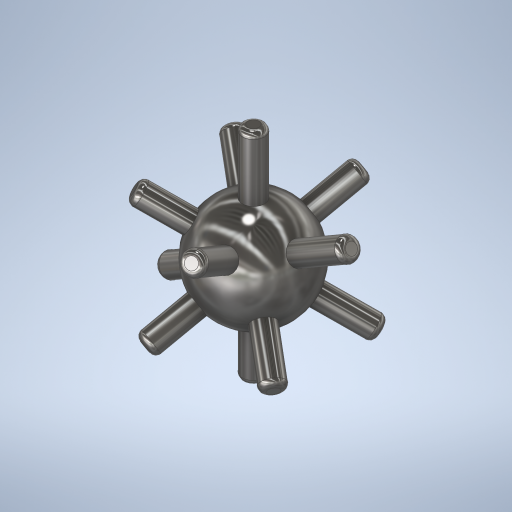
# Autodesk Inventor part: jezek v
Saved by Autodesk Inventor 2023 (Build 270158000, 158)
## iProperties
Created: 2024-01-23
Part Number: jezek v
Material: Všeobecné
Document SubType Name: Modeling
Designer: 42073
Density: 1 g/cm^3
Appearance: Ocel – leštěná
Mass: 5.1124 g
Surface Area: 25.3749 cm^2
Volume: 5.1124 cm^3
Author: 42073
Autodesk Inventor part; units mm, degrees
sketch "Náčrt1" plane through (0, 0, 0) normal (0, 0, 1) x (1, 0, 0)
  circle A0 centre (0, 0) radius 9.6
  dimension "d0" = 19.2
  constraints: 1 centre point, 1 coincident
  measures "d0" diameter of A0
extrude "Vysunutí1" add sketch "Náčrt1" along normal mid plane 19.2
fillet "Zaoblení1" radius 9.6 2 edges at (-9.6, 0, 9.6) (-9.6, 0, -9.6)
sketch "Náčrt2" plane through (0, 0, 0) normal (0, 0, 1) x (1, 0, 0)
  line L0 (0, 0) -> (20, 0)
  line L1 (0, 0) -> (6.1803, 19.0211)
  line L2 (0, 0) -> (20, 0) construction
  line L3 (0, 0) -> (-16.1803, 11.7557)
  line L4 (0, 0) -> (20, 0) construction
  line L5 (0, 0) -> (-16.1803, -11.7557)
  line L6 (0, 0) -> (20, 0) construction
  line L7 (0, 0) -> (6.1803, -19.0211)
  line L8 (0, 0) -> (20, 0) construction
  dimension "d4" = 20
  dimension "d5" = 20
  dimension "d6" = 72
  dimension "d7" = 20
  dimension "d8" = 144
  dimension "d9" = 20
  dimension "d10" = 216
  dimension "d11" = 20
  dimension "d12" = 72
  constraints: 18 end point, 5 horizontal, 4 equal length
  measures "d4" distance of L0.start L0.end
  measures "d5" distance of L0.start L1.end
  measures "d6" angle of L2 L1
  measures "d7" distance of L0.start L3.end
  measures "d8" angle of L4 L3
  measures "d9" distance of L0.start L5.end
  measures "d11" distance of L0.start L7.end
  measures "d12" angle of L7 L8
ref_plane "Pracovní rovina2" through (0, 0, 20) normal (0, 0, 1) x (1, 0, 0)
sketch "Náčrt3" plane through (0, 0, 20) normal (0, 0, 1) x (1, 0, 0)
  line L0 (0, 0) -> (6.1803, 19.0211)
  line L1 (0, 0) -> (20, 0) construction
  line L2 (0, 0) -> (-16.1803, 11.7557)
  line L3 (0, 0) -> (20, 0) construction
  line L4 (0, 0) -> (20, 0)
  line L5 (0, 0) -> (6.1803, -19.0211)
  line L6 (0, 0) -> (20, 0) construction
  line L7 (0, 0) -> (-16.1803, -11.7557)
  line L8 (0, 0) -> (20, 0) construction
  dimension "d14" = 20
  dimension "d15" = 72
  dimension "d16" = 20
  dimension "d17" = 144
  dimension "d18" = 20
  dimension "d19" = 72
  dimension "d20" = 20
  dimension "d21" = 144
  constraints: 18 end point, 4 equal length, 4 horizontal, 1 collinear
  measures "d14" distance of L0.start L0.end
  measures "d15" angle of L1 L0
  measures "d16" distance of L0.start L2.end
  measures "d17" angle of L3 L2
  measures "d18" distance of L0.start L5.end
  measures "d19" angle of L5 L6
  measures "d20" distance of L0.start L7.end
  measures "d21" angle of L7 L8
ref_plane "Pracovní rovina3" through (0, 0, 20) normal (-0.9511, 0.309, 0) x (0.309, 0.9511, 0)
sketch "Náčrt4" plane through (0, 0, 20) normal (-0.9511, 0.309, 0) x (0.309, 0.9511, 0)
  line L0 (0, 20) -> (0, 39.1)
  line L1 (0, 20) -> (15.9349, 10.8)
  line L2 (0, 20) -> (18.4, 20) construction
  line L3 (0, 20) -> (-15.7617, 29.1)
  line L4 (0, 20) -> (0, -1.1)
  dimension "d22" = 19.1
  dimension "d23" = 18.4
  dimension "d24" = 30
  dimension "d25" = 18.2
  dimension "d26" = 21.1
  constraints: 10 end point, 2 vertical, 1 equal length, 1 horizontal, 1 point on line
  measures "d22" distance of L0.start L0.end
  measures "d23" distance of L0.start L1.end
  measures "d24" angle of L1 L2
  measures "d25" distance of L0.start L3.end
  measures "d26" distance of L0.start L4.end
ref_plane "Pracovní rovina4" through (0, 0, 0) normal (0, -1, 0) x (1, 0, 0)
sketch "Náčrt5" plane through (0, 0, 0) normal (0, -1, 0) x (1, 0, 0)
  line L0 (0, 0) -> (17.9267, 10.35)
  line L1 (0, 0) -> (20.7, 0) construction
  line L2 (0, 0) -> (-15.9349, -9.2)
  dimension "d27" = 20.7
  dimension "d28" = 30
  dimension "d29" = 18.4
  constraints: 6 end point, 1 equal length, 1 horizontal
  measures "d27" distance of L0.start L0.end
  measures "d28" angle of L1 L0
  measures "d29" distance of L0.start L2.end
ref_plane "Pracovní rovina5" through (0, 0, 0) normal (-0.9511, -0.309, 0) x (0.309, -0.9511, 0)
sketch "Náčrt6" plane through (0, 0, 0) normal (-0.9511, -0.309, 0) x (0.309, -0.9511, 0)
  line L0 (0, 0) -> (17.6669, 10.2)
  line L1 (0, 0) -> (20.4, 0) construction
  line L2 (0, 0) -> (-16.5411, -9.55)
  dimension "d30" = 20.4
  dimension "d31" = 30
  dimension "d32" = 19.1
  constraints: 6 end point, 1 equal length, 1 horizontal
  measures "d30" distance of L0.start L0.end
  measures "d31" angle of L1 L0
  measures "d32" distance of L0.start L2.end
ref_plane "Pracovní rovina6" through (0, 0, 20) normal (0.5878, -0.809, 0) x (-0.809, -0.5878, 0)
sketch "Náčrt7" plane through (0, 0, 20) normal (0.5878, -0.809, 0) x (-0.809, -0.5878, 0)
  line L0 (0, 20) -> (15.6751, 10.95)
  line L1 (0, 20) -> (18.1, 20) construction
  line L2 (0, 20) -> (-16.6277, 29.6)
  dimension "d33" = 18.1
  dimension "d34" = 30
  dimension "d35" = 19.2
  constraints: 6 end point, 1 equal length, 1 horizontal
  measures "d33" distance of L0.start L0.end
  measures "d34" angle of L0 L1
  measures "d35" distance of L0.start L2.end
ref_plane "Pracovní rovina7" through (0, 0, 0) normal (0.5878, 0.809, 0) x (-0.809, 0.5878, 0)
sketch "Náčrt8" plane through (0, 0, 0) normal (0.5878, 0.809, 0) x (-0.809, 0.5878, 0)
  line L0 (0, 0) -> (16.3679, 9.45)
  line L1 (0, 0) -> (18.9, 0) construction
  line L2 (0, 0) -> (-16.6277, -9.6)
  dimension "d36" = 18.9
  dimension "d37" = 30
  dimension "d38" = 19.2
  constraints: 6 end point, 1 equal length, 1 horizontal, 1 point on line
  measures "d36" distance of L0.start L0.end
  measures "d37" angle of L1 L0
  measures "d38" distance of L0.start L2.end
ref_plane "Pracovní rovina8" through (0, 0, 21.1) normal (0, 0, 1) x (1, 0, 0)
ref_plane "Pracovní rovina9" through (0, 0, -19.1) normal (0, 0, -1) x (-1, 0, 0)
sketch "Náčrt9" plane through (0, 0, 21.1) normal (0, 0, 1) x (1, 0, 0)
  circle A0 centre (0, 0) radius 2
  dimension "d39" = 4
  constraints: 1 centre point, 1 coincident
  measures "d39" diameter of A0
sketch "Náčrt10" plane through (0, 0, -19.1) normal (0, 0, -1) x (-1, 0, 0)
  circle A0 centre (0, 0) radius 2
  dimension "d40" = 4
  constraints: 1 centre point, 1 coincident
  measures "d40" diameter of A0
extrude "Vysunutí2" add sketch "Náčrt9" against normal up to surface
extrude "Vysunutí3" add sketch "Náčrt10" against normal up to surface
ref_plane "Pracovní rovina10" through (-12.6814, -9.2136, 9.05) normal (-0.7006, -0.509, 0.5) x (0.5878, -0.809, 0)
ref_plane "Pracovní rovina11" through (13.4521, 9.7735, -9.6) normal (0.7006, 0.509, -0.5) x (-0.5878, 0.809, 0)
sketch "Náčrt11" plane through (-12.6814, -9.2136, 9.05) normal (-0.7006, -0.509, 0.5) x (0.5878, -0.809, 0)
  circle A0 centre (0, 0) radius 2
  dimension "d45" = 4
  constraints: 1 centre point, 1 coincident
  measures "d45" diameter of A0
sketch "Náčrt12" plane through (13.4521, 9.7735, -9.6) normal (0.7006, 0.509, -0.5) x (-0.5878, 0.809, 0)
  circle A0 centre (0, 0) radius 2
  dimension "d46" = 4
  constraints: 1 centre point, 1 coincident
  measures "d46" diameter of A0
extrude "Vysunutí4" add sketch "Náčrt12" against normal up to surface
extrude "Vysunutí5" add sketch "Náčrt11" against normal up to surface
ref_plane "Pracovní rovina12" through (-13.2419, 9.6208, 9.45) normal (-0.7006, 0.509, 0.5) x (-0.5878, -0.809, 0)
ref_plane "Pracovní rovina13" through (13.4521, -9.7735, -9.6) normal (0.7006, -0.509, -0.5) x (0.5878, 0.809, 0)
sketch "Náčrt13" plane through (-13.2419, 9.6208, 9.45) normal (-0.7006, 0.509, 0.5) x (-0.5878, -0.809, 0)
  circle A0 centre (0, 0) radius 2
  dimension "d51" = 4
  constraints: 1 centre point, 1 coincident
  measures "d51" diameter of A0
sketch "Náčrt14" plane through (13.4521, -9.7735, -9.6) normal (0.7006, -0.509, -0.5) x (0.5878, 0.809, 0)
  circle A0 centre (0, 0) radius 2
  dimension "d52" = 4
  constraints: 1 centre point, 1 coincident
  measures "d52" diameter of A0
extrude "Vysunutí6" add sketch "Náčrt14" against normal up to surface
extrude "Vysunutí7" add sketch "Náčrt13" against normal up to surface
ref_plane "Pracovní rovina14" through (-5.1115, 15.7315, -9.55) normal (-0.2676, 0.8236, -0.5) x (-0.9511, -0.309, 0)
ref_plane "Pracovní rovina15" through (5.4594, -16.8022, 10.2) normal (0.2676, -0.8236, 0.5) x (0.9511, 0.309, 0)
sketch "Náčrt15" plane through (-5.1115, 15.7315, -9.55) normal (-0.2676, 0.8236, -0.5) x (-0.9511, -0.309, 0)
  circle A0 centre (0, 0) radius 2
  dimension "d57" = 4
  constraints: 1 centre point, 1 coincident
  measures "d57" diameter of A0
sketch "Náčrt16" plane through (5.4594, -16.8022, 10.2) normal (0.2676, -0.8236, 0.5) x (0.9511, 0.309, 0)
  circle A0 centre (0, 0) radius 2
  dimension "d58" = 4
  constraints: 1 centre point, 1 coincident
  measures "d58" diameter of A0
extrude "Vysunutí8" add sketch "Náčrt15" against normal up to surface
extrude "Vysunutí9" add sketch "Náčrt16" against normal up to surface
ref_plane "Pracovní rovina16" through (4.9241, 15.155, 9.2) normal (0.2676, 0.8236, 0.5) x (-0.9511, 0.309, 0)
ref_plane "Pracovní rovina17" through (-4.8706, -14.9902, -9.1) normal (-0.2676, -0.8236, -0.5) x (0.9511, -0.309, 0)
sketch "Náčrt17" plane through (4.9241, 15.155, 9.2) normal (0.2676, 0.8236, 0.5) x (-0.9511, 0.309, 0)
  circle A0 centre (0, 0) radius 2
  dimension "d63" = 4
  constraints: 1 centre point, 1 coincident
  measures "d63" diameter of A0
sketch "Náčrt18" plane through (-4.8706, -14.9902, -9.1) normal (-0.2676, -0.8236, -0.5) x (0.9511, -0.309, 0)
  circle A0 centre (0, 0) radius 2
  dimension "d64" = 4
  constraints: 1 centre point, 1 coincident
  measures "d64" diameter of A0
extrude "Vysunutí10" add sketch "Náčrt17" against normal up to surface
extrude "Vysunutí11" add sketch "Náčrt18" against normal up to surface
ref_plane "Pracovní rovina18" through (17.9267, 0, 10.35) normal (0.866, 0, 0.5) x (0, 1, 0)
ref_plane "Pracovní rovina19" through (-15.9349, 0, -9.2) normal (-0.866, 0, -0.5) x (0, -1, 0)
sketch "Náčrt19" plane through (17.9267, 0, 10.35) normal (0.866, 0, 0.5) x (0, 1, 0)
  circle A0 centre (0, 0) radius 2
  dimension "d69" = 4
  constraints: 1 centre point, 1 coincident
  measures "d69" diameter of A0
sketch "Náčrt20" plane through (-15.9349, 0, -9.2) normal (-0.866, 0, -0.5) x (0, -1, 0)
  circle A0 centre (0, 0) radius 2
  dimension "d70" = 4
  constraints: 1 centre point, 1 coincident
  measures "d70" diameter of A0
extrude "Vysunutí12" add sketch "Náčrt20" against normal up to surface
extrude "Vysunutí13" add sketch "Náčrt19" against normal up to surface
sketch "Náčrt21" plane through (17.9267, 0, 10.35) normal (0.866, 0, 0.5) x (0, 1, 0)
  circle A0 centre (0, 0) radius 2
  dimension "d75" = 4
  constraints: 1 centre point, 1 coincident
  measures "d75" diameter of A0
sketch "Náčrt22" plane through (-15.9349, 0, -9.2) normal (-0.866, 0, -0.5) x (0, -1, 0)
  circle A0 centre (0, 0) radius 2
  dimension "d76" = 4
  constraints: 1 centre point, 1 coincident
  measures "d76" diameter of A0
extrude "Vysunutí14" cut sketch "Náčrt21" against normal blind 0.221
extrude "Vysunutí15" cut sketch "Náčrt22" against normal blind 0.221
sketch "Náčrt23" plane through (4.9241, 15.155, 9.2) normal (0.2676, 0.8236, 0.5) x (-0.9511, 0.309, 0)
  circle A0 centre (0, 0) radius 2
  dimension "d81" = 4
  constraints: 1 centre point, 1 coincident
  measures "d81" diameter of A0
sketch "Náčrt24" plane through (-4.8706, -14.9902, -9.1) normal (-0.2676, -0.8236, -0.5) x (0.9511, -0.309, 0)
  circle A0 centre (0, 0) radius 2
  dimension "d82" = 4
  constraints: 1 centre point, 1 coincident
  measures "d82" diameter of A0
extrude "Vysunutí16" cut sketch "Náčrt23" against normal blind 0.221
extrude "Vysunutí17" cut sketch "Náčrt24" against normal blind 0.221
sketch "Náčrt25" plane through (5.4594, -16.8022, 10.2) normal (0.2676, -0.8236, 0.5) x (0.9511, 0.309, 0)
  circle A0 centre (0, 0) radius 2
  dimension "d87" = 4
  constraints: 1 centre point, 1 coincident
  measures "d87" diameter of A0
sketch "Náčrt26" plane through (-5.1115, 15.7315, -9.55) normal (-0.2676, 0.8236, -0.5) x (-0.9511, -0.309, 0)
  circle A0 centre (0, 0) radius 2
  dimension "d88" = 4
  constraints: 1 centre point, 1 coincident
  measures "d88" diameter of A0
extrude "Vysunutí18" cut sketch "Náčrt25" against normal blind 0.221
extrude "Vysunutí19" cut sketch "Náčrt26" against normal blind 0.221
sketch "Náčrt27" plane through (-13.2419, 9.6208, 9.45) normal (-0.7006, 0.509, 0.5) x (-0.5878, -0.809, 0)
  circle A0 centre (0, 0) radius 2
  dimension "d93" = 4
  constraints: 1 centre point, 1 coincident
  measures "d93" diameter of A0
sketch "Náčrt28" plane through (13.4521, -9.7735, -9.6) normal (0.7006, -0.509, -0.5) x (0.5878, 0.809, 0)
  circle A0 centre (0, 0) radius 2
  dimension "d94" = 4
  constraints: 1 centre point, 1 coincident
  measures "d94" diameter of A0
extrude "Vysunutí20" cut sketch "Náčrt27" against normal blind 0.221
extrude "Vysunutí21" cut sketch "Náčrt28" against normal blind 0.221
sketch "Náčrt29" plane through (-12.6814, -9.2136, 9.05) normal (-0.7006, -0.509, 0.5) x (0.5878, -0.809, 0)
  circle A0 centre (0, 0) radius 2
  dimension "d99" = 4
  constraints: 1 centre point, 1 coincident
  measures "d99" diameter of A0
sketch "Náčrt30" plane through (13.4521, 9.7735, -9.6) normal (0.7006, 0.509, -0.5) x (-0.5878, 0.809, 0)
  circle A0 centre (0, 0) radius 2
  dimension "d100" = 4
  constraints: 1 centre point, 1 coincident
  measures "d100" diameter of A0
extrude "Vysunutí22" cut sketch "Náčrt30" against normal blind 0.221
extrude "Vysunutí23" cut sketch "Náčrt29" against normal blind 0.221
sketch "Náčrt31" plane through (0, 0, -19.1) normal (0, 0, -1) x (-1, 0, 0)
  circle A0 centre (0, 0) radius 2
  dimension "d105" = 4
  constraints: 1 centre point, 1 coincident
  measures "d105" diameter of A0
sketch "Náčrt32" plane through (0, 0, 21.1) normal (0, 0, 1) x (1, 0, 0)
  circle A0 centre (0, 0) radius 2
  dimension "d106" = 4
  constraints: 1 centre point, 1 coincident
  measures "d106" diameter of A0
extrude "Vysunutí24" cut sketch "Náčrt31" against normal blind 0.221
extrude "Vysunutí25" cut sketch "Náčrt32" against normal blind 0.221
fillet "Zaoblení2" radius 1 12 edges at (3.4976, -17.2366, 10.0885) (-13.7007, -7.482, 8.9385) (-2, 0, 20.879) (-6.7131, -14.1885, -8.9885) (12.1203, -11.278, -9.4885) (2, 0, -18.879) (14.4714, 8.042, -9.4885) (-3.1497, 16.1659, -9.4385) (6.7666, 14.3533, 9.0885) (-11.9101, 11.1253, 9.3385) (17.7336, -2, 10.2385) (-15.7417, 2, -9.0885)
